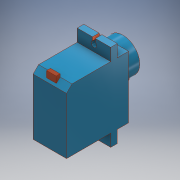
# Autodesk Inventor part: SG92r
Saved by Autodesk Inventor 2018 (Build 220112000, 112)
## iProperties
Created: 2020-10-02
Part Number: SG92r
Material: Ogólny
Document SubType Name: Modeling
Designer: Raven
Density: 1 g/cm^3
Appearance: Gorący metal 1400F
Author: Raven
Autodesk Inventor part; units mm, degrees
ref_plane "YZ Plane" through (0, 0, 0) normal (1, 0, 0) x (0, 1, 0)
ref_plane "XZ Plane" through (0, 0, 0) normal (0, 1, 0) x (-1, 0, 0)
ref_plane "XY Plane" through (0, 0, 0) normal (0, 0, 1) x (1, 0, 0)
sketch "Szkic1" plane through (0, 0, 0) normal (0, 1, 0) x (-1, 0, 0)
  line L0 (0, 0) -> (12.2, 0)
  line L1 (12.2, 0) -> (12.2, -22.6)
  line L2 (12.2, -22.6) -> (0, -22.6)
  line L3 (0, -22.6) -> (0, 0)
  dimension "d0" = 12.2
  dimension "d1" = 22.6
  constraints: 8 end point, 2 parallel, 1 horizontal, 1 perpendicular
  measures "d0" distance of L1.end L2.end
  measures "d1" distance of L0.end L1.end
extrude "Wyciągnięcie proste1" add sketch "Szkic1" along normal blind 22.6
sketch "Szkic2" plane through (-12.2, 0, 0) normal (0, 0, 1) x (1, 0, 0)
  line L0 (0, 22.6) -> (12.2, 22.6) construction
  line L1 (0, 22.6) -> (0, 18.5) construction
  line L2 (0, 0) -> (0, 22.6) construction
  line L3 (0, 18.5) -> (12.2, 18.5) construction
  line L4 (12.2, 0) -> (12.2, 22.6) construction
  line L5 (0, 18.5) -> (0, 16.1) construction
  line L6 (0, 18.5) -> (12.2, 18.5)
  line L7 (12.2, 18.5) -> (12.2, 16.1)
  line L8 (12.2, 16.1) -> (0, 16.1)
  line L9 (0, 16.1) -> (0, 18.5)
  dimension "d4" = 4.1
  dimension "d5" = 2.4
  constraints: 14 end point, 4 point on line, 2 parallel, 2 perpendicular, 1 horizontal
  measures "d4" distance of L0.start L1.end
  measures "d5" distance of L1.end L5.end
extrude "Wyciągnięcie proste2" add sketch "Szkic2" along normal blind 4.5
sketch "Szkic3" plane through (0, 0, -22.6) normal (0, 0, -1) x (-1, 0, 0)
  line L0 (12.2, 18.5) -> (0, 18.5) projected
  line L1 (0, 16.1) -> (12.2, 16.1) projected
  line L2 (12.2, 0) -> (12.2, 22.6) projected
  line L3 (0, 0) -> (0, 22.6) projected
  line L4 (12.2, 18.5) -> (0, 18.5)
  line L5 (0, 18.5) -> (0, 16.1)
  line L6 (0, 16.1) -> (12.2, 16.1)
  line L7 (12.2, 16.1) -> (12.2, 18.5)
  constraints: 8 end point, 2 parallel, 1 horizontal, 1 perpendicular
extrude "Wyciągnięcie proste3" add sketch "Szkic3" along normal blind 4.5
sketch "Szkic4" plane through (-12.2, 18.5, 0) normal (0, 1, 0) x (1, 0, 0)
  line L0 (0, -4.5) -> (12.2, -4.5) construction
  line L1 (6.1, -4.5) -> (6.1, 27) construction
  line L2 (6.1, -4.5) -> (5.6, -4.5) construction
  line L3 (6.1, -4.5) -> (6.1, -2.4) construction
  circle A0 centre (6.1, -2.4) radius 1 construction
  line L4 (5.6, -4.5) -> (6.6, -4.5) construction
  line L5 (6.6, -4.5) -> (6.6, -3) construction
  line L6 (6.6, -3) -> (5.6, -3) construction
  line L7 (5.6, -3) -> (5.6, -4.5) construction
  line L8 (5.6, -4.5) -> (5.6, -3.266)
  line L9 (5.6, -4.5) -> (6.6, -4.5)
  line L10 (6.6, -4.5) -> (6.6, -3.266)
  arc A1 (6.6, -3.266) -> (5.6, -3.266) centre (6.1, -2.4) ccw
  line L11 (0, 22.6) -> (0, 0) construction
  line L12 (0, 11.3) -> (12.2, 11.3) construction
  line L13 (12.2, 0) -> (12.2, 22.6) construction
  circle A2 centre (6.1, 25) radius 1 construction
  line L14 (5.6, 27.1) -> (6.6, 27.1) construction
  line L15 (5.6, 27.1) -> (5.6, 25.866)
  line L16 (6.6, 27.1) -> (6.6, 25.866)
  line L17 (5.6, 27.1) -> (6.6, 27.1)
  line L18 (0, 27.1) -> (12.2, 27.1) projected
  arc A3 (5.6, 25.866) -> (6.6, 25.866) centre (6.1, 25) ccw
  dimension "d10" = 0.5
  dimension "d11" = 2.1
  dimension "d12" = 2
  dimension "d13" = 1
  constraints: 30 end point, 8 point on circle, 5 symmetric about line, 4 centre point, 4 point on line, 3 midpoint, 2 collinear, 2 parallel, 1 coincident, 1 horizontal, 1 perpendicular, 1 vertical, 1 other
  measures "d10" distance of L1.start L2.end
  measures "d11" distance of L1.start L3.end
  measures "d12" diameter of A0
  measures "d13" distance of L6.end L5.end
extrude "Wyciągnięcie proste4" cut sketch "Szkic4" against normal blind 2.4
sketch "Szkic5" plane through (0, 22.6, 0) normal (0, 1, 0) x (1, 0, 0)
  line L0 (-12.2, 0) -> (0, 0) construction
  line L1 (-6.1, 0) -> (-6.1, 6.1) construction
  circle A0 centre (-6.1, 6.1) radius 6.1 construction
  line L2 (-6.1, 0) -> (-6.1, 14.5) construction
  circle A1 centre (-6.1, 12.2) radius 2.3 construction
  arc A2 (-8.3588, 11.7664) -> (-3.8412, 11.7664) centre (-6.1, 6.1) ccw
  arc A3 (-3.8412, 11.7664) -> (-8.3588, 11.7664) centre (-6.1, 12.2) ccw
  dimension "d16" = 6.1
  dimension "d17" = 12.2
  dimension "d18" = 14.5
  constraints: 12 point on circle, 4 centre point, 4 end point, 2 point on line, 1 coincident, 1 midpoint, 1 vertical
  measures "d16" distance of L1.start L1.end
  measures "d17" diameter of A0
  measures "d18" distance of L1.start L2.end
extrude "Wyciągnięcie proste5" add sketch "Szkic5" along normal blind 4.1
sketch "Szkic6" plane through (0, 26.7, 0) normal (0, 1, 0) x (1, 0, 0)
  arc A0 (-8.3588, 11.7664) -> (-3.8412, 11.7664) centre (-6.1, 6.1) ccw projected
  circle A1 centre (-6.1, 6.1) radius 2.4
  point P0 (0, 0)
  dimension "d21" = 4.8
  constraints: 1 centre point, 1 coincident
  measures "d21" diameter of A1
extrude "Wyciągnięcie proste6" add sketch "Szkic6" along normal blind 2.6
chamfer "Faza1" distance 2 angle 45 1 edges at (-6.1, 0, 0)
sketch "Szkic7" plane through (-12.2, 16.1, 0) normal (0, 0, 1) x (1, 0, 0)
  line L0 (12.2, -14.1) -> (0, -14.1) construction
  line L1 (6.1, -14.1) -> (6.1, -16.1) construction
  line L2 (0, -16.1) -> (12.2, -16.1) construction
  line L3 (6.1, -14.1) -> (4.35, -14.1) construction
  line L4 (4.35, -14.1) -> (7.85, -14.1)
  line L5 (7.85, -14.1) -> (7.85, -15.5)
  line L6 (7.85, -15.5) -> (4.35, -15.5)
  line L7 (4.35, -15.5) -> (4.35, -14.1)
  dimension "d27" = 1.75
  dimension "d28" = 3.5
  dimension "d29" = 1.4
  constraints: 12 end point, 2 midpoint, 2 parallel, 2 perpendicular, 1 horizontal
  measures "d27" distance of L1.start L3.end
  measures "d28" distance of L5.end L6.end
  measures "d29" distance of L4.end L5.end
extrude "Wyciągnięcie proste7" add sketch "Szkic7" along normal blind 1 and the other way blind 1.3
